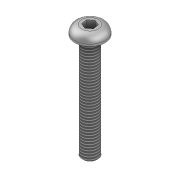
# Autodesk Inventor part: Tornillo Allen cabeeza botón M3x20mm
Saved by Autodesk Inventor 2020 (Build 240168000, 168)
## iProperties
Created: 2020-05-08
Part Number: Tornillo Allen cabeeza botón M3x20mm
Material: Generic
Document SubType Name: Modeling
Designer: Dante
Density: 1 g/cm^3
Appearance: Rubber - Black - Version 1.1
Mass: 0.335505 g
Surface Area: 3.39406 cm^2
Volume: 0.335505 cm^3
Author: Dante
Autodesk Inventor part; units mm, degrees
ref_plane "YZ Plane" through (0, 0, 0) normal (1, 0, 0) x (0, 1, 0)
ref_plane "XZ Plane" through (0, 0, 0) normal (0, 1, 0) x (-1, 0, 0)
ref_plane "XY Plane" through (0, 0, 0) normal (0, 0, 1) x (1, 0, 0)
sketch "Sketch1" plane through (0, 0, 0) normal (0, 0, 1) x (1, 0, 0)
  line L0 (-10.627, -30.5907) -> (-13.477, -30.5907)
  line L1 (-10.627, -30.5907) -> (-10.627, -50.5907)
  line L2 (-10.627, -50.5907) -> (-12.127, -50.5907)
  line L3 (-12.127, -50.5907) -> (-12.127, -30.5907)
  line L4 (-10.627, -30.5907) -> (-10.627, -26.5988)
  line L5 (-13.477, -30.5907) -> (-13.477, -30.2107)
  line L6 (-13.477, -30.2107) -> (-13.477, -28.9407)
  line L7 (-13.477, -28.9407) -> (-10.627, -28.9407)
  dimension "d0" = 2.85
  dimension "d2" = 20
  dimension "d3" = 1.5
  dimension "d18" = 0.38
  dimension "d19" = 1.65
  constraints: 16 end point, 3 point on line, 3 vertical, 2 horizontal, 2 perpendicular
  measures "d0" distance of L0.start L0.end
  measures "d2" distance of L0.start L1.end
  measures "d3" distance of L1.end L2.end
  measures "d18" distance of L0.end L5.end
  measures "d19" distance between parallel lines of L0 L7
revolve "Revolution1" add sketch "Sketch1" angle 360 about axis through (-10.627, -30.5907, 0) along (0, -1, 0)
chamfer "Chamfer2" distance 0.2 angle 45 1 edges at (-9.127, -50.5907, 0)
fillet "Empalme2" radius 1.27 1 edges at (-7.777, -28.9407, 0)
sketch "Boceto2" plane through (-10.627, -28.9407, 0) normal (0, 1, 0) x (1, 0, 0)
  line L0 (0.8985, 0.7252) -> (1.0773, -0.4156)
  line L1 (1.0773, -0.4156) -> (0.1788, -1.1408)
  line L2 (0.1788, -1.1408) -> (-0.8985, -0.7252)
  line L3 (-0.8985, -0.7252) -> (-1.0773, 0.4156)
  line L4 (-1.0773, 0.4156) -> (-0.1788, 1.1408)
  line L5 (-0.1788, 1.1408) -> (0.8985, 0.7252)
  point P0 (10.627, 0)
  point P1 (0, 0)
  dimension "d21" = 2
  constraints: 12 end point, 13 other
  measures "d21" distance between parallel lines of L1 L4
extrude "Extrusión1" cut sketch "Boceto2" against normal blind 1.3
thread "Rosca2" size "M3x0.5" class "6g" standard "ISO Metric profile" length 430
body "Solid1"
